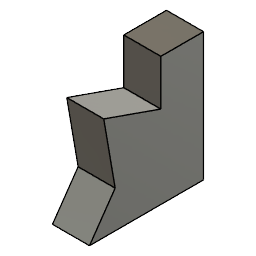
replay (Autodesk Fusion 360 design; units mm, degrees)
Autodesk Fusion 360 part; units mm, degrees
ref_plane "工作平面1" through (17, 0, 0) normal (1, 0, 0) x (0, 1, 0)
sketch "草图1" plane through (17, 0, 0) normal (1, 0, 0) x (0, 0, -1)
  line L0 (-5, 35) -> (-20, 35)
  line L1 (-20, 35) -> (-20, 19)
  line L2 (-20, 19) -> (-40, 26)
  line L3 (-40, 26) -> (-36, 3)
  line L4 (-36, 3) -> (-45, -10)
  line L5 (-45, -10) -> (-5, -10)
  line L6 (-5, -10) -> (-5, 35)
extrude "拉伸1" add sketch "草图1" along normal blind 13
